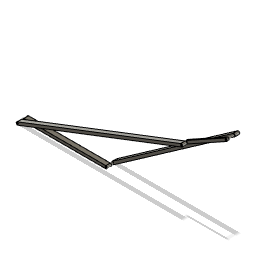
ME21B005_ProjectAnimation (Autodesk Fusion 360 design; units mm, degrees)
Autodesk Fusion 360 part; units mm, degrees
sketch "Sketch1" plane through (0, 0, 0) normal (0, 1, 0) x (1, 0, 0)
sketch "Sketch2" plane through (0, 0, 0) normal (0, 0, 1) x (1, 0, 0)
  line L0 (0, 0) -> (49.71, 0) construction
  line L1 (43.4773, 24.0999) -> (207.3873, 24.0999) construction
  line L2 (42.617, 25.3286) -> (-91.6502, -68.6863)
  line L3 (44.3377, 22.8712) -> (-89.9295, -71.1438)
  circle A0 centre (-90.7899, -69.915) radius 0.75
  circle A1 centre (43.4773, 24.0999) radius 0.75
  arc A2 (44.3377, 22.8712) -> (42.617, 25.3286) centre (43.4773, 24.0999) ccw
  arc A3 (-91.6502, -68.6863) -> (-89.9295, -71.1438) centre (-90.7899, -69.915) ccw
  line L4 (-181.2514, -71.3151) -> (0.5384, -1.4)
  line L5 (-182.3283, -68.515) -> (-0.5384, 1.4)
  circle A4 centre (-181.7899, -69.915) radius 0.75
  circle A5 centre (0, 0) radius 0.75
  arc A6 (0.5384, -1.4) -> (-0.5384, 1.4) centre (0, 0) ccw
  arc A7 (-182.3283, -68.515) -> (-181.2514, -71.3151) centre (-181.7899, -69.915) ccw
  dimension "d2" = 49.71
  dimension "d5" = 91
  dimension "d16" = 1.5
  dimension "d17" = 1.5
  dimension "d29" = 1.5
  dimension "d30" = 1.5
  constraint horizontal L0
  constraint horizontal L1
  constraint tangent L2 A3
  constraint concentric A0 A3
  constraint coincident L1.start A1.centre
  constraint tangent L2 A2
  constraint concentric A1 A2
  constraint tangent L5 A7
  constraint coincident L0.start A5.centre
  constraint tangent L5 A6
  constraint concentric A5 A6
  measures "d2" distance of L0.start L1.start
  measures "d5" distance of A0.centre A4.centre
  measures "d16" diameter of A0
  measures "d17" diameter of A1
  measures "d29" diameter of A4
  measures "d30" diameter of A5
sketch "Sketch3" plane through (0, 0, 0) normal (0, 0, 1) x (1, 0, 0)
sketch "Sketch4" plane through (0, 0, 0) normal (0, 0, 1) x (1, 0, 0)
  line L0 (100, 0) -> (149.71, 0) construction
  line L1 (100.7272, -1.3119) -> (144.2046, 22.788)
  line L2 (99.2728, 1.3119) -> (142.7501, 25.4118)
  circle A0 centre (100, 0) radius 0.75
  circle A1 centre (143.4773, 24.0999) radius 0.75
  arc A2 (99.2728, 1.3119) -> (100.7272, -1.3119) centre (100, 0) ccw
  arc A3 (144.2046, 22.788) -> (142.7501, 25.4118) centre (143.4773, 24.0999) ccw
  dimension "d6" = 49.71
  dimension "d10" = 1.5
  dimension "d11" = 1.5
  constraint horizontal L0
  constraint coincident L0.start A0.centre
  constraint tangent L2 A2
  constraint concentric A0 A2
  constraint tangent L2 A3
  measures "d6" distance of L0.start A1.centre
  measures "d10" diameter of A0
  measures "d11" diameter of A1
extrude "Extrude1" add sketch "Sketch4" along normal blind 2 makes body 1
sketch "Sketch5" plane through (0, 0, 0) normal (0, 0, 1) x (1, 0, 0)
extrude "Extrude2" add sketch "Sketch2" along normal blind 5 separate body contours L2 L3 A2 A3 makes body 2
copy_body "Body->Comp1" bodies 1 removing the originals makes body 3 in component "Component"
copy_body "Body->Comp2" bodies 2 removing the originals makes body 4 in component "Component'"
sketch "Sketch6" plane through (0, 0, 0) normal (0, 0, 1) x (1, 0, 0)
  line L0 (120, 1.5) -> (29, 1.5)
  line L1 (120, -1.5) -> (29, -1.5)
  circle A0 centre (120, 0) radius 0.75
  circle A1 centre (29, 0) radius 0.75
  arc A2 (29, 1.5) -> (29, -1.5) centre (29, 0) ccw
  arc A3 (120, -1.5) -> (120, 1.5) centre (120, 0) ccw
  dimension "d20" = 91
  dimension "d23" = 1.5
  dimension "d24" = 1.5
  constraint tangent L0 A2
  constraint tangent L0 A3
  constraint concentric A0 A3
  constraint concentric A1 A2
  measures "d20" distance of A1.centre A0.centre
  measures "d23" diameter of A0
  measures "d24" diameter of A1
extrude "Extrude3" add sketch "Sketch6" along normal blind 5 separate body makes body 5
copy_body "Body->Comp3" bodies 5 removing the originals makes body 6 in component "Component''"
extrude "Extrude4" add sketch "Sketch2" along normal blind 5 separate body contours L4 L5 A6 A7 makes body 7
sketch "Sketch7" plane through (0, 0, 0) normal (0, 0, 1) x (1, 0, 0)
  circle A0 centre (-20, 10) radius 0.75
  circle A1 centre (-16, 12) radius 0.75
  circle A2 centre (-13, 13) radius 0.75
  circle A3 centre (-28, 12) radius 0.75
  dimension "d33" = 1.5
  dimension "d34" = 1.5
  dimension "d35" = 1.5
  dimension "d36" = 1.5
  measures "d33" diameter of A0
  measures "d34" diameter of A1
  measures "d35" diameter of A2
  measures "d36" diameter of A3
extrude "Extrude5" add sketch "Sketch7" along normal blind 15 separate body contours A3 makes body 8
extrude "Extrude6" add sketch "Sketch7" along normal blind 15 separate body contours A0 | A1 | A2 makes body 9 at (-20.3422, 10.6674, 10) makes body 10 at (-16.3422, 12.6674, 10) makes body 11 at (-12.2537, 12.9253, 10)
copy_body "Body->Comp4" bodies 7 removing the originals makes body 12 in component "Component'''"
copy_body "Body->Comp5" bodies 8 removing the originals makes body 13 in component "Component''''"
copy_body "Body->Comp6" bodies 9 removing the originals makes body 14 in component "Component'''''"
copy_body "Body->Comp7" bodies 10 removing the originals makes body 15 in component "Component''''''"
copy_body "Body->Comp8" bodies 11 removing the originals makes body 16 in component "Component'''''''"
move_face "OffsetFaces1" offset 5 1 faces at (-13.1437, 13.4658, 0) on bodies 16 in component "Component'''''''"
move_face "OffsetFaces1'" offset -7 1 faces at (-15.9059, 11.8045, 0) on bodies 15 in component "Component''''''"
move_face "OffsetFaces1''" offset -3 1 faces at (-27.8195, 12.1328, 0) on bodies 13 in component "Component''''"
move_face "OffsetFaces1'''" offset -3 1 faces at (-19.8195, 10.1328, 0) on bodies 14 in component "Component'''''"
move_face "OffsetFaces2" offset -6 1 faces at (-13.2252, 12.8915, 15) on bodies 16 in component "Component'''''''"
component "Component" placed x (1, 0, 0) y (0, 1, 0) z (0, 0, 1) at (-100, 0, -3)
component "Component'" placed x (1, 0.00003, 0) y (-0.00003, 1, 0) z (0, 0, 1) at (0.0007, -0.0013, -15)
component "Component''" placed x (1, 0.000036, 0) y (-0.000036, 1, 0) z (0, 0, 1) at (-210.7871, -69.9234, -7)
component "Component'''" placed x (1, 0.00004, 0) y (-0.00004, 1, 0) z (0, 0, 1) at (0, 0, 0)
component "Component''''" placed x (1, 0.000036, 0) y (-0.000036, 1, 0) z (0, 0, 1) at (-153.7866, -81.9213, -10)
component "Component'''''" placed x (1, 0.00003, 0) y (-0.00003, 1, 0) z (0, 0, 1) at (-70.7868, -79.9184, -18)
component "Component''''''" placed x (1, 0, 0) y (0, 1, 0) z (0, 0, 1) at (16, -12, -10)
component "Component'''''''" placed x (1, 0, 0) y (0, 1, 0) z (0, 0, 1) at (56.4773, 11.0999, -10)
